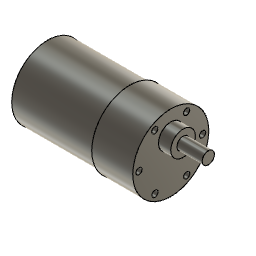
motor raspberry pi mount (Autodesk Fusion 360 archive; units mm, degrees)
design "Motor"
Autodesk Fusion 360 part; units mm, degrees
sketch "Sketch1" plane through (0, 0, 0) normal (1, 0, 0) x (0, 1, 0)
  circle A0 centre (0, 0) radius 17.5
  line L0 (0, 0) -> (0, 17.5)
  dimension "d1" = 35
  constraint coincident A0.centre L0.start
  constraint coincident A0 L0.end
  measures "d1" diameter of A0
extrude "Extrude1" add sketch "Sketch1" along normal blind 40
sketch "Sketch2" plane through (40, 0, 0) normal (1, 0, 0) x (0, 1, 0)
  circle A0 centre (0, 0) radius 17.5
  circle A1 centre (0, 0) radius 18.5
  point P0 (0, 7)
  dimension "d5" = 37
  constraint coincident A0.centre A1.centre
  measures "d5" diameter of A1
extrude "Extrude2" add sketch "Sketch2" along normal blind 20 contours A0 | A1
sketch "Sketch3" plane through (60, 0, 0) normal (1, 0, 0) x (0, 1, 0)
  circle A0 centre (0, 0) radius 18.5
  line L0 (0, 0) -> (0, 7)
  circle A1 centre (0, 7) radius 6
  circle A2 centre (0, 0) radius 15.5 construction
  line L1 (0, 0) -> (0, 15.5)
  circle A3 centre (-15.4999, -0.0425) radius 1.5
  circle A4 centre (-7.7132, -13.4446) radius 1.5
  circle A5 centre (7.7868, -13.4021) radius 1.5
  circle A6 centre (15.4999, 0.0425) radius 1.5
  circle A7 centre (7.7132, 13.4446) radius 1.5
  circle A8 centre (-7.7868, 13.4021) radius 1.5
  dimension "d8" = 12
  dimension "d9" = 31
  dimension "d10" = 3
  dimension "d12" = 360
  constraint coincident A0.centre L0.start
  constraint vertical L0
  constraint coincident L0.end A1.centre
  constraint coincident A2 L1.end
  constraint parallel L0 L1
  constraint coincident A2 A3.centre
  measures "d8" diameter of A1
  measures "d9" diameter of A2
  measures "d10" diameter of A3
extrude "Extrude3" cut sketch "Sketch3" against normal blind 3 contours A3 | A4 | A5 | A6 | A7 | A8
sketch "Sketch4" plane through (60, 0, 0) normal (1, 0, 0) x (0, 1, 0)
  circle A0 centre (7.7868, -13.4021) radius 1.5
  circle A1 centre (-7.7868, 13.4021) radius 1.5
  circle A2 centre (15.4999, 0.0425) radius 1.5
  circle A3 centre (-7.7132, -13.4446) radius 1.5
  circle A4 centre (-15.4999, -0.0425) radius 1.5
  circle A5 centre (7.7132, 13.4446) radius 1.5
  circle A6 centre (0, 0) radius 18.5
  circle A7 centre (0, 0) radius 18.5
  line L0 (0, 0) -> (0, 7) construction
  circle A8 centre (0, 7) radius 6
  dimension "d15" = 37
  dimension "d16" = 7
  dimension "d17" = 12
  constraint coincident A6.centre A7.centre
  constraint vertical L0
  constraint coincident L0.end A8.centre
  measures "d15" diameter of A7
  measures "d16" distance of A6.centre L0.end
  measures "d17" diameter of A8
extrude "Extrude4" add sketch "Sketch4" along normal blind 6 contours A8
sketch "Sketch6" plane through (66, 0, 0) normal (1, 0, 0) x (0, 1, 0)
  circle A0 centre (0, 7) radius 6
  circle A1 centre (0, 7) radius 3
  dimension "d21" = 6
  constraint concentric A0 A1
  measures "d21" diameter of A1
extrude "Extrude5" add sketch "Sketch6" along normal blind 12.3 contours A1
